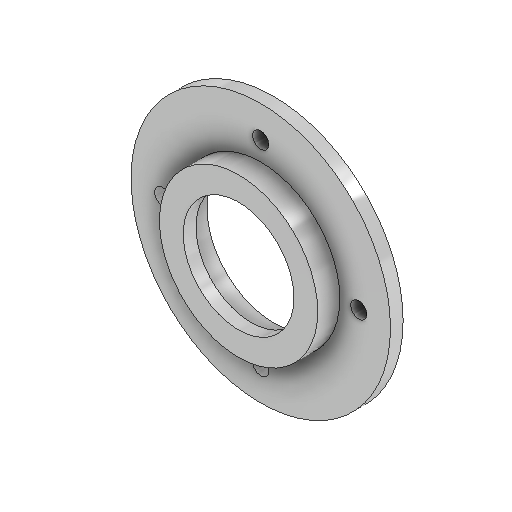
# Autodesk Inventor part: BearingHolder
Saved by Autodesk Inventor 2022 (Build 260153000, 153)
## iProperties
Created: 2024-07-02
Part Number: BearingHolder
Material: Generic
Document SubType Name: Modeling
Designer: LaptopJR
Density: 1 g/cm^3
Appearance: Aluminum - Polished
Author: LaptopJR
Autodesk Inventor part; units mm, degrees
ref_plane "YZ Plane" through (0, 0, 0) normal (1, 0, 0) x (0, 1, 0)
ref_plane "XZ Plane" through (0, 0, 0) normal (0, 1, 0) x (-1, 0, 0)
ref_plane "XY Plane" through (0, 0, 0) normal (0, 0, 1) x (1, 0, 0)
sketch "Sketch1" plane through (0, 0, 0) normal (0, 0, 1) x (1, 0, 0)
  circle A0 centre (0, 0) radius 21
  circle A1 centre (0, 0) radius 41
  circle A2 centre (0, 0) radius 31 construction
  circle A3 centre (0, 31) radius 2.55
  circle A4 centre (-31, 0) radius 2.55
  circle A5 centre (0, -31) radius 2.55
  circle A6 centre (31, 0) radius 2.55
  dimension "d0" = 42
  dimension "d1" = 20
  dimension "d2" = 10
  dimension "d3" = 5.1
  dimension "d6" = 360
  constraints: 6 centre point, 3 coincident, 1 vertical alignment, 11 other
  measures "d0" diameter of A0
  measures "d1" radial gap between concentric circles of A1 A0
  measures "d3" diameter of A3
extrude "Extrusion1" add sketch "Sketch1" along normal blind 4
sketch "Sketch2" plane through (0, 0, 4) normal (0, 0, 1) x (1, 0, 0)
  circle A0 centre (0, 0) radius 25
  circle A1 centre (0, 0) radius 21 projected
  dimension "d10" = 4
  constraints: 1 centre point, 1 coincident
  measures "d10" radial gap between concentric circles of A0 A1
extrude "Extrusion2" add sketch "Sketch2" along normal blind 3
sketch "Sketch3" plane through (0, 0, 7) normal (0, 0, 1) x (1, 0, 0)
  circle A0 centre (0, 0) radius 25 projected
  circle A1 centre (0, 0) radius 17.5
  dimension "d13" = 35
  constraints: 1 centre point, 1 coincident
  measures "d13" diameter of A1
extrude "Extrusion3" add sketch "Sketch3" along normal blind 4
body "Solid1"
